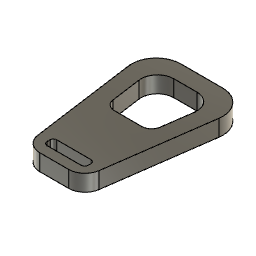
Upptakari (Autodesk Fusion 360 design; units mm, degrees)
Autodesk Fusion 360 part; units mm, degrees
sketch "Sketch1" plane through (0, 0, 0) normal (0, 0, 1) x (1, 0, 0)
  line L0 (18.6978, -81.3757) -> (27.6301, -17.0635)
  line L1 (12.7727, 0) -> (-12.7727, 0)
  line L2 (-27.6301, -17.0635) -> (-18.6978, -81.3757)
  line L3 (-8.7929, -90) -> (8.7929, -90)
  arc A0 (-12.7727, 0) -> (-27.6301, -17.0635) centre (-12.7727, -15) ccw
  arc A1 (27.6301, -17.0635) -> (12.7727, 0) centre (12.7727, -15) ccw
  arc A2 (-18.6978, -81.3757) -> (-8.7929, -90) centre (-8.7929, -80) ccw
  arc A3 (8.7929, -90) -> (18.6978, -81.3757) centre (8.7929, -80) ccw
  line L4 (10.5, -78) -> (-10.5, -78)
  line L5 (-12.5, -80) -> (-12.5, -82)
  line L6 (-10.5, -84) -> (10.5, -84)
  line L7 (12.5, -82) -> (12.5, -80)
  arc A4 (-10.5, -78) -> (-12.5, -80) centre (-10.5, -80) ccw
  arc A5 (12.5, -80) -> (10.5, -78) centre (10.5, -80) ccw
  arc A6 (-12.5, -82) -> (-10.5, -84) centre (-10.5, -82) ccw
  arc A7 (10.5, -84) -> (12.5, -82) centre (10.5, -82) ccw
  line L8 (14.3727, -39.8254) -> (16.9352, -21.3757)
  line L9 (7.0302, -10) -> (-7.0302, -10)
  line L10 (-16.9352, -21.3757) -> (-14.3727, -39.8254)
  line L11 (-8.4297, -45) -> (8.4297, -45)
  arc A8 (-7.0302, -10) -> (-16.9352, -21.3757) centre (-7.0302, -20) ccw
  arc A9 (16.9352, -21.3757) -> (7.0302, -10) centre (7.0302, -20) ccw
  arc A10 (8.4297, -45) -> (14.3727, -39.8254) centre (8.4297, -39) ccw
  arc A11 (-14.3727, -39.8254) -> (-8.4297, -45) centre (-8.4297, -39) ccw
  point P0 (17.5, -90)
  point P1 (30, 0)
  point P2 (-30, 0)
  point P3 (-17.5, -90)
  point P4 (12.5, -78)
  point P5 (-12.5, -78)
  point P6 (12.5, -84)
  dimension "d3" = 90
  dimension "d4" = 60
  dimension "d5" = 35
  dimension "d9" = 12.5
  dimension "d10" = 15
  dimension "d11" = 15
  dimension "d12" = 10
  dimension "d13" = 10
  dimension "d14" = 25
  dimension "d15" = 6
  dimension "d16" = 6
  dimension "d17" = 2
  dimension "d18" = 2
  dimension "d19" = 2
  dimension "d20" = 2
  dimension "d21" = 12.5
  dimension "d22" = 10
  dimension "d23" = 10
  dimension "d24" = 6
  dimension "d25" = 6
  dimension "d26" = 10
  dimension "d27" = 10
  dimension "d28" = 10
  dimension "d29" = 35
  constraint horizontal L1
  constraint horizontal L3
  constraint coincident P2 L1
  constraint coincident P2 L2
  constraint tangent L1 A0
  constraint tangent L2 A0
  constraint coincident P1 L1
  constraint coincident P1 L0
  constraint tangent L1 A1
  constraint tangent L0 A1
  constraint coincident P3 L2
  constraint coincident P3 L3
  constraint tangent L2 A2
  constraint tangent L3 A2
  constraint coincident P0 L0
  constraint coincident P0 L3
  constraint tangent L0 A3
  constraint tangent L3 A3
  constraint horizontal L4
  constraint vertical L5
  constraint horizontal L6
  constraint vertical L7
  constraint coincident P5 L4
  constraint coincident P5 L5
  constraint tangent L4 A4
  constraint tangent L5 A4
  constraint coincident P4 L4
  constraint coincident P4 L7
  constraint tangent L4 A5
  constraint tangent L7 A5
  constraint tangent L5 A6
  constraint tangent L6 A6
  constraint coincident P6 L7
  constraint coincident P6 L6
  constraint tangent L7 A7
  constraint tangent L6 A7
  constraint midpoint origin L1
  constraint horizontal L9
  constraint parallel L9 L11
  constraint tangent L9 A8
  constraint tangent L10 A8
  constraint tangent L9 A9
  constraint tangent L8 A9
  constraint tangent L8 A10
  constraint tangent L11 A10
  constraint tangent L10 A11
  constraint tangent L11 A11
  constraint parallel L0 L8
  constraint parallel L2 L10
  measures "d3" distance of L1 L3
  measures "d4" distance of P1 P2
  measures "d5" distance of P0 P3
  measures "d9" horizontal distance of P0 P1
  measures "d10" radius of A0
  measures "d11" radius of A1
  measures "d12" radius of A2
  measures "d13" radius of A3
  measures "d14" distance of P4 P5
  measures "d15" distance of P4 P6
  measures "d16" distance of L3 L6
  measures "d17" radius of A4
  measures "d18" radius of A5
  measures "d19" radius of A6
  measures "d20" radius of A7
  measures "d21" horizontal distance of origin L7.start
  measures "d22" radius of A8
  measures "d23" radius of A9
  measures "d24" radius of A10
  measures "d25" radius of A11
  measures "d26" distance of L1 L9
  measures "d27" distance of L0 L8
  measures "d28" distance of L2 L10
  measures "d29" distance of L9 L11
extrude "Extrude1" add sketch "Sketch1" along normal blind 15
extrude "Extrude2" cut 1 faces at (2.8099, -67, 15) along direction (0, 0, -1) blind 3
extrude "Extrude3" cut 1 faces at (2.8099, -67, 12) along direction (0, 0, -1) blind 2
sketch "Sketch2" plane through (0, -45, 0) normal (0, 1, 0) x (-1, 0, 0)
  line L0 (8.4297, 10) -> (-8.4297, 10)
  line L1 (-8.4297, 10) -> (-8.4297, 0)
  line L2 (-8.4297, 0) -> (8.4297, 0)
  line L3 (8.4297, 0) -> (8.4297, 10)
  line L4 (12.5, 5.75) -> (-12.5, 5.75)
  line L5 (-12.5, 5.75) -> (-12.5, 4.25)
  line L6 (-12.5, 4.25) -> (12.5, 4.25)
  line L7 (12.5, 4.25) -> (12.5, 5.75)
  point P0 (-12.7727, 10)
  dimension "d36" = 25
  dimension "d37" = 1.5
  dimension "d38" = 12.5
  dimension "d39" = 4.25
  constraint horizontal L4
  constraint vertical L5
  constraint horizontal L6
  constraint vertical L7
  measures "d36" horizontal distance of L4.end L6.end
  measures "d37" distance of L4.start L6
  measures "d38" horizontal distance of origin L4.start
  measures "d39" vertical distance of L4.end P0
extrude "Extrude4" cut sketch "Sketch2" along normal blind 3 and the other way blind 15 contours L3 L4 L6 L7 | L1 L3 L4 L6 | L1 L4 L5 L6
sketch "Sketch3" plane through (0, 0, 10) normal (0, 0, 1) x (-1, 0, 0)
  arc A0 (-10.5, 84) -> (-12.5, 82) centre (-10.5, 82) ccw
  line L0 (-10.5, 84) -> (10.5, 84)
  arc A1 (12.5, 82) -> (10.5, 84) centre (10.5, 82) ccw
  line L1 (12.5, 82) -> (12.5, 80)
  arc A2 (10.5, 78) -> (12.5, 80) centre (10.5, 80) ccw
  line L2 (10.5, 78) -> (-10.5, 78)
  arc A3 (-12.5, 80) -> (-10.5, 78) centre (-10.5, 80) ccw
  line L3 (-12.5, 80) -> (-12.5, 82)
  arc A4 (14.3727, 39.8254) -> (8.4297, 45) centre (8.4297, 39) ccw
  line L4 (14.3727, 39.8254) -> (16.9352, 21.3757)
  arc A5 (7.0302, 10) -> (16.9352, 21.3757) centre (7.0302, 20) ccw
  line L5 (7.0302, 10) -> (-7.0302, 10)
  arc A6 (-16.9352, 21.3757) -> (-7.0302, 10) centre (-7.0302, 20) ccw
  line L6 (-16.9352, 21.3757) -> (-14.3727, 39.8254)
  arc A7 (-8.4297, 45) -> (-14.3727, 39.8254) centre (-8.4297, 39) ccw
  line L7 (-8.4297, 45) -> (8.4297, 45)
  arc A8 (-8.7929, 90) -> (-18.6978, 81.3757) centre (-8.7929, 80) ccw
  line L8 (-18.6978, 81.3757) -> (-27.6301, 17.0635)
  arc A9 (-27.6301, 17.0635) -> (-12.7727, 0) centre (-12.7727, 15) ccw
  line L9 (-12.7727, 0) -> (12.7727, 0)
  arc A10 (12.7727, 0) -> (27.6301, 17.0635) centre (12.7727, 15) ccw
  line L10 (27.6301, 17.0635) -> (18.6978, 81.3757)
  arc A11 (18.6978, 81.3757) -> (8.7929, 90) centre (8.7929, 80) ccw
  line L11 (8.7929, 90) -> (-8.7929, 90)
equation "D_krona = 25 mm"
equation "þykkt_krona = 1.5 mm"
equation "d3 = haed"
equation "d4 = max_b"
equation "d5 = min_b"
equation "max_b = 60 mm"
equation "min_b = 35 mm"
equation "haed = 90 mm"
equation "d9 = ( max_b - min_b ) / 2"
equation "d14 = D_krona"
equation "d21 = D_krona / 2"
equation "d36 = D_krona"
equation "d37 = þykkt_krona"
equation "d38 = D_krona / 2"
equation "d39 = ( 10 mm - þykkt_krona ) / 2"
equation "d42 = D_krona - 10 mm"
